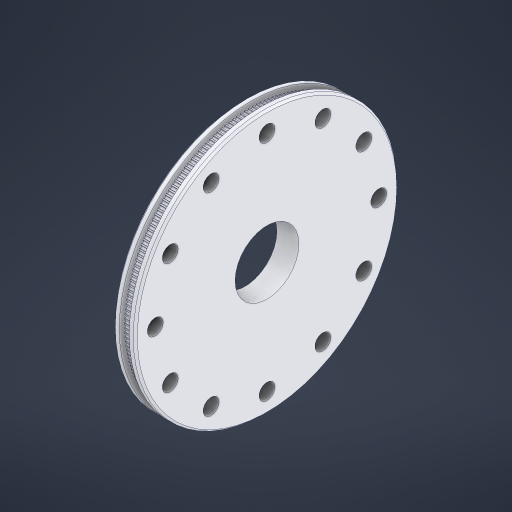
# Autodesk Inventor part: TurretPulley
Saved by Autodesk Inventor 2024 (Build 280153000, 153)
## iProperties
Created: 2023-10-25
Part Number: TurretPulley
Material: Generic
Document SubType Name: Modeling
Designer: avsar
Density: 1 g/cm^3
Appearance: PTFE
Author: avsar
Autodesk Inventor part; units mm, degrees
ref_plane "YZ Plane" through (0, 0, 0) normal (1, 0, 0) x (0, 1, 0)
ref_plane "XZ Plane" through (0, 0, 0) normal (0, 1, 0) x (-1, 0, 0)
ref_plane "XY Plane" through (0, 0, 0) normal (0, 0, 1) x (1, 0, 0)
sketch "Sketch1" plane through (0, 0, 0) normal (1, 0, 0) x (0, 1, 0)
  circle A0 centre (0, 0) radius 63.408 construction
  circle A1 centre (0, 0) radius 62.658 construction
  line L0 (0, 0) -> (63.408, 0) construction
  line L1 (0, 0) -> (0, -63.408) construction
  circle A2 centre (63.213, 0) radius 0.555 construction
  line L2 (0, 0) -> (63.3767, -1.9917) construction
  circle A3 centre (63.1818, -1.9856) radius 0.555 construction
  circle A4 centre (63.2541, -0.7038) radius 0.15 construction
  circle A5 centre (63.245, -1.2834) radius 0.15 construction
  arc A6 (62.658, 0) -> (63.2453, -0.5541) centre (63.213, 0) ccw
  arc A7 (63.4041, -0.7055) -> (63.2453, -0.5541) centre (63.2541, -0.7038) ccw
  arc A8 (63.3949, -1.2864) -> (63.4041, -0.7055) centre (0, 0) ccw
  arc A9 (63.2315, -1.4328) -> (63.3949, -1.2864) centre (63.245, -1.2834) ccw
  arc A10 (63.2315, -1.4328) -> (62.6271, -1.9681) centre (63.1818, -1.9856) ccw
  arc A11 (62.6271, -1.9681) -> (62.658, 0) centre (0, 0) ccw
  dimension "d0" = 126.816
  dimension "d1" = -0.75
  dimension "d2" = 1.11
  dimension "d4" = 88.2
  dimension "d5" = 0.3
  constraints: 25 point on circle, 12 centre point, 8 equal radius, 8 tangent, 6 end point, 4 point on line, 1 coincident, 1 concentric, 1 horizontal, 1 perpendicular
  measures "d0" diameter of A0
  measures "d1" radial gap between concentric circles of A0 A1
  measures "d2" diameter of A2
  measures "d4" angle of L1 L2
  measures "d5" diameter of A4
extrude "Extrusion1" add sketch "Sketch1" along normal mid plane 5
pattern_circular "Circular Pattern1" count 200 over 360 about axis through (-10, 0, 0) along (1, 0, 0) of "Extrusion1"
sketch "Sketch2" plane through (0, 0, 0) normal (1, 0, 0) x (0, 1, 0)
  arc A0 (62.6271, 1.9681) -> (63.2315, 1.4328) centre (63.1818, 1.9856) ccw projected
  circle A1 centre (0, 0) radius 62.658
  constraints: 1 coincident, 3 other
extrude "Extrusion2" add sketch "Sketch2" along normal mid plane 5
sketch "Sketch4" plane through (2.5, 0, 0) normal (1, 0, 0) x (0, 0, -1)
  circle A0 centre (0, 0) radius 66
  dimension "d14" = 132
  constraints: 1 centre point, 1 coincident
  measures "d14" diameter of A0
extrude "Extrusion3" add sketch "Sketch4" along normal blind 3
sketch "Sketch5" plane through (-2.5, 0, 0) normal (-1, 0, 0) x (0, 0, 1)
  circle A0 centre (0, 0) radius 66 projected
extrude "Extrusion4" add sketch "Sketch5" along normal blind 3
chamfer "Chamfer1" distance 1 angle 45 2 edges at (-5.5, 0, -66) (5.5, 0, 66)
sketch "Sketch6" plane through (5.5, 0, 0) normal (1, 0, 0) x (0, 0, -1)
  circle A0 centre (0, 0) radius 16
  circle A1 centre (0, 56) radius 4
  circle A2 centre (-28, 48.4974) radius 4
  circle A3 centre (-48.4974, 28) radius 4
  circle A4 centre (-56, 0) radius 4
  circle A5 centre (-48.4974, -28) radius 4
  circle A6 centre (-28, -48.4974) radius 4
  circle A7 centre (0, -56) radius 4
  circle A8 centre (28, -48.4974) radius 4
  circle A9 centre (48.4974, -28) radius 4
  circle A10 centre (56, 0) radius 4
  circle A11 centre (48.4974, 28) radius 4
  circle A12 centre (28, 48.4974) radius 4
  dimension "d22" = 32
  dimension "d23" = 8
  dimension "d24" = 56
  dimension "d27" = 360
  constraints: 13 centre point, 1 coincident, 1 vertical alignment, 25 other
  measures "d22" diameter of A0
  measures "d23" diameter of A1
  measures "d24" distance of point (0, 0) A1.centre
extrude "Extrusion5" cut sketch "Sketch6" against normal through all
equation "\"d0\" = OD_"
equation "\"d1\" = H_"
equation "\"d2\" = BTD_"
equation "\"d4\" = TH_"
equation "\"d5\" = PTR_"
equation "\"d6\" = EX_"
equation "\"d11\" = EX_"
equation "\"U_\" = 0.254"
equation "\"H_\" = -0.75"
equation "\"P_\" = 2"
equation "\"BTD_\" = 1.11"
equation "\"PTR_\" = 0.3"
equation "\"EX_\" = 5"
equation "\"OD_\" = PD_ - 2 * U_"
equation "\"TH_\" = 88.2deg"
equation "\"PD_\" = 127.323954"
body "Solid1"
